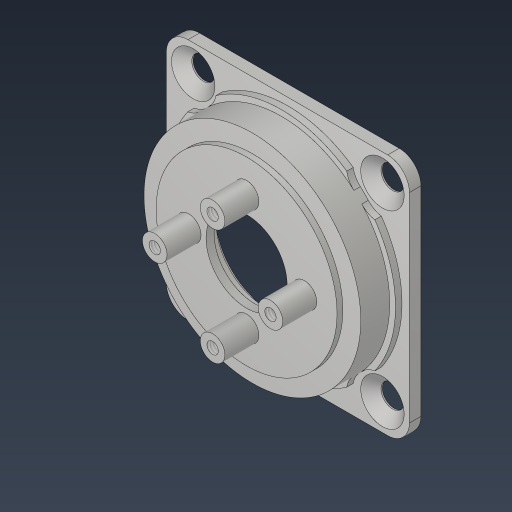
# Autodesk Inventor part: Getriebe Planetenhalter
Saved by Autodesk Inventor 2023.1 (Build 271208000, 208)
## iProperties
Part Number: Getriebe Planetenhalter
Material: Aluminium 6061
Document SubType Name: Modeling
Designer: rYan
Mass: 8.99181 g
Surface Area: 33.1784 cm^2
Volume: 3.3303 cm^3
Density: 2.7 g/cm^3
Appearance: Aluminium - flach
Author: rYan
Autodesk Inventor part; units mm, degrees
ref_plane "YZ Plane" through (0, 0, 0) normal (1, 0, 0) x (0, 1, 0)
ref_plane "XZ Plane" through (0, 0, 0) normal (0, 1, 0) x (-1, 0, 0)
ref_plane "XY Plane" through (0, 0, 0) normal (0, 0, 1) x (1, 0, 0)
sketch "Skizze1" plane through (0, 0, 0) normal (0, 0, 1) x (1, 0, 0)
  line L0 (0, 0) -> (0, 7.3)
  line L1 (14.98, 7.3) -> (14.98, 0.8)
  line L2 (5.6, 0) -> (5.6, 2.5)
  line L3 (7.45, 3.2) -> (13.5, 3.2)
  line L4 (13.5, 3.2) -> (13.5, 7.3)
  line L5 (13.5, 7.3) -> (14.98, 7.3)
  line L6 (12.5, 0) -> (5.6, 0)
  line L7 (7.45, 3.2) -> (7.45, 2.5)
  line L8 (7.45, 2.5) -> (5.6, 2.5)
  line L9 (12.5, 0) -> (12.5, 0.8)
  line L10 (12.5, 0.8) -> (14.98, 0.8)
  point P0 (0, 3.65)
  dimension "d4" = 11.2
  dimension "d5" = 4.1
  dimension "d6" = 27
  dimension "d24" = 14.9
  dimension "d25" = 0.7
  dimension "d63" = 29.96
  dimension "d64" = 1.48
  dimension "d79" = 25
  dimension "d82" = 6.5
  dimension "d83" = 0.8
  constraints: 22 end point, 6 perpendicular, 4 vertical, 2 point on line, 1 midpoint
  measures "d4" diameter of L2 L0
  measures "d5" distance of L3.end L4.end
  measures "d6" diameter of L4 L0
  measures "d24" diameter of L7 L0
  measures "d25" distance of L3.start L7.end
  measures "d63" diameter of L1 L0
  measures "d64" distance between parallel lines of L4 L1
  measures "d79" diameter of L9 L0
  measures "d82" distance between parallel lines of L10 L5
  measures "d83" distance from line of L0.start L10
revolve "Umdrehung1" add sketch "Skizze1" angle 360 about axis through (0, 0, 0) along (0, 1, 0)
sketch "Skizze8" plane through (0, 0, 0) normal (0, -1, 0) x (1, 0, 0)
  line L0 (0, 20.972) -> (0, -20.972) construction
  circle A0 centre (0, 8) radius 1.7
  point P0 (0, 0)
  dimension "d65" = 3.4
  dimension "d66" = 8
  constraints: 1 centre point, 1 point on line
  measures "d65" diameter of A0
  measures "d66" distance of point (0, 0) A0.centre
extrude "Extrusion5" add sketch "Skizze8" along normal blind 4.7
sketch "Skizze9" plane through (0, -4.7, 8) normal (0, -1, 0) x (1, 0, 0)
  circle A0 centre (0, 0) radius 1.7 projected
  point P0 (0, -8)
  constraints: 1 coincident
hole "Bohrung3" at (0, -4.7, 8) direction (0, 1, 0) diameter 1.567 end through all thread size "M2x0.4" class "6H" standard "ISO Metric profile"
sketch "Skizze12" plane through (0, 2.5, 0) normal (0, 1, 0) x (1, 0, 0)
  arc A0 (-0.5381, -7.4305) -> (0.5381, -7.4305) centre (0, -8) ccw construction
  circle A1 centre (0, -8) radius 1.55
  point P0 (0, 0)
  dimension "d92" = 3.1
  constraints: 1 centre point, 1 coincident
  measures "d92" diameter of A1
extrude "Extrusion7" cut sketch "Skizze12" along normal through all
fillet "Rundung3" radius 1 2 edges at (-1.3923, 2.85, 7.3188) (1.3923, 2.85, 7.3188)
pattern_circular "Runde Anordnung3" count 4 over 360 about axis through (0, -10, 0) along (0, 1, 0) of "Extrusion5", "Bohrung3", "Extrusion7", "Rundung3"
sketch "Skizze3" plane through (0, 7.3, 0) normal (0, 1, 0) x (1, 0, 0)
  line L0 (16.8, -16.8) -> (-16.8, -16.8)
  line L1 (-16.8, -16.8) -> (-16.8, 16.8)
  line L2 (-16.8, 16.8) -> (16.8, 16.8)
  line L3 (16.8, 16.8) -> (16.8, -16.8)
  line L4 (16.8, -16.8) -> (-16.8, 16.8) construction
  line L5 (-16.8, -16.8) -> (16.8, 16.8) construction
  circle A0 centre (0, 0) radius 13.5 projected
  point P0 (0, 0)
  dimension "d28" = 33.6
  dimension "d29" = 33.6
  constraints: 12 end point, 2 midpoint, 2 parallel, 1 horizontal, 1 perpendicular
  measures "d28" distance of L1.end L2.end
  measures "d29" distance of L0.end L1.end
extrude "Extrusion1" add sketch "Skizze3" against normal blind 1.6
sketch "Skizze4" plane through (0, 5.7, 0) normal (0, -1, 0) x (1, 0, 0)
  circle A0 centre (0, 0) radius 18.5 construction
  line L0 (-13.0815, 13.0815) -> (13.0815, -13.0815) construction
  line L1 (13.0815, 13.0815) -> (-13.0815, -13.0815) construction
  line L2 (0, 25.9) -> (0, -25.9) construction
  point P0 (0, 0)
  dimension "d32" = 37
  constraints: 5 coincident, 4 end point, 4 point on circle, 3 midpoint, 1 centre point, 1 perpendicular, 1 other
  measures "d32" diameter of A0
hole "Bohrung2" at (-13.0815, 5.7, 13.0815) at (13.0815, 5.7, 13.0815) at (13.0815, 5.7, -13.0815) at (-13.0815, 5.7, -13.0815) direction (0, 1, 0) diameter 3.2 end through all countersink diameter 6 countersink angle 90
fillet "Rundung1" radius 3 4 edges at (16.8, 6.5, 16.8) (-16.8, 6.5, 16.8) (-16.8, 6.5, -16.8) (16.8, 6.5, -16.8)
sketch "Skizze5" plane through (-13.8, 7.3, -16.8) normal (0, 1, 0) x (1, 0, 0)
  circle A0 centre (13.8, -16.8) radius 11 construction
  line L0 (13.8, 6.72) -> (13.8, -40.32) construction
  circle A1 centre (13.8, -5.8) radius 3.2
  dimension "d41" = 22
  dimension "d42" = 6.4
  constraints: 1 centre point, 1 coincident, 1 point on line, 1 vertical alignment, 2 other
  measures "d42" diameter of A1
extrude "Extrusion2" cut sketch "Skizze5" against normal blind 1.4
pattern_circular "Runde Anordnung2" count 3 over 360 about axis through (0, -10, 0) along (0, 1, 0) of "Extrusion2"
sketch "Skizze6" plane through (-13.8, 7.3, -16.8) normal (0, 1, 0) x (1, 0, 0)
  line L0 (13.8, 6.72) -> (13.8, -40.32) construction
  circle A0 centre (8.3, -28.8) radius 2.5
  circle A1 centre (19.3, -28.8) radius 2.5
  point P0 (13.8, -16.8)
  dimension "d48" = 5.5
  dimension "d49" = 12
  dimension "d50" = 5
  constraints: 2 centre point, 1 other
  measures "d48" horizontal distance of A0.centre point (13.8, -16.8)
  measures "d49" vertical distance of A0.centre point (13.8, -16.8)
  measures "d50" diameter of A0
extrude "Extrusion3" cut sketch "Skizze6" against normal blind 1.4
sketch "Skizze10" plane through (0, 5.7, 0) normal (0, -1, 0) x (1, 0, 0)
  circle A0 centre (0, 0) radius 14.98 projected
  circle A1 centre (0, 0) radius 15.78
  line L0 (0, 0) -> (9.051, 12.9262)
  line L1 (0, 0) -> (-9.051, 12.9262)
  line L2 (0, 23.52) -> (0, -23.52) construction
  point P0 (-8.5922, 12.2709)
  point P1 (8.5922, 12.2709)
  dimension "d84" = 0.8
  dimension "d85" = 70
  constraints: 4 end point, 2 point on circle, 1 centre point, 1 coincident, 1 other
  measures "d84" radial gap between concentric circles of A1 A0
  measures "d85" angle of L0 L1
extrude "Extrusion6" add sketch "Skizze10" along normal blind 0.9 contours A0 L1 A1 L0 picked at (-0.6085, 15.3977)
fillet "Rundung2" radius 3.1 2 edges at (-8.5922, 5.25, 12.2709) (8.5922, 5.25, 12.2709)
pattern_circular "Runde Anordnung4" count 4 over 360 about axis through (0, -10, 0) along (0, 1, 0) of "Extrusion6", "Rundung2"
sketch "Skizze13" plane through (0, 2.5, 8) normal (0, 1, 0) x (1, 0, 0)
  circle A0 centre (0, 8) radius 5.6 projected
  circle A1 centre (0, 8) radius 6.7
  dimension "d96" = 13.4
  constraints: 1 centre point, 1 coincident
  measures "d96" diameter of A1
extrude "Extrusion8" cut sketch "Skizze13" against normal blind 1.4
